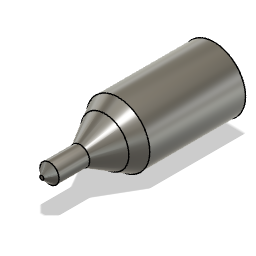
ME contact pin v2 (Autodesk Fusion 360 design; units mm, degrees)
Autodesk Fusion 360 part; units mm, degrees
sketch "Sketch1" plane through (0, 0, 0) normal (0, 1, 0) x (1, 0, 0)
  line L0 (0, 0) -> (0, -9)
  line L1 (0, -9) -> (0.5, -9)
  line L2 (0.5, -9) -> (0.5, 0)
  line L3 (0.5, -7) -> (1.65, -5.0081)
  line L4 (1.65, -5.0081) -> (1.65, 0)
  line L5 (1.65, 0) -> (0, 0)
  line L6 (1.25, 0) -> (1.25, -5.701)
  dimension "d1" = 0.5
  dimension "d2" = 9
  dimension "d3" = 2
  dimension "d4" = 0.75
  dimension "d5" = 0.4
  dimension "d6" = 30
  constraint coincident L0.start L5.end
  constraint vertical L0
  constraint perpendicular L0 L1
  constraint perpendicular L1 L2
  constraint parallel L0 L4
  constraint perpendicular L0 L5
  constraint coincident L5 L6.start
  constraint coincident L3 L6.end
  constraint perpendicular L5 L6
  constraint coincident L5 L2.end
  constraint coincident L3.start L2
  measures "d1" distance of L0.end L1.end
  measures "d2" distance of L0.start L0.end
  measures "d3" distance of L1.end L3.start
  measures "d4" distance of L2 L6
  measures "d5" distance of L4 L6
  measures "d6" angle of L2 L3
revolve "Revolve1" add sketch "Sketch1" angle 360 about axis through (0, 0, 0) along (0, 0, 1) contours L0 L1 L2 L5 makes body 1
revolve "Revolve2" add sketch "Sketch1" angle 360 about axis through (0, 0, 9) along (0, 0, -1) separate body contours L2 L3 L5 L6 makes body 2
revolve "Revolve3" add sketch "Sketch1" angle 360 about axis through (0, 0, 0) along (0, 0, 1) separate body contours L3 L4 L5 L6 makes body 3
chamfer "Chamfer1" distance 0.4 angle 45 1 edges at (-0.4662, -0.1808, 9) on bodies 1
